Autodesk Inventor part; units mm, degrees
(part 2 of 2)
  line L261 (-632.3012, 486.9524) -> (-657.7012, 472.2877)
  arc A340 (-632.3012, 486.9524) -> (-632.3012, 495.7513) centre (-634.8412, 491.3518) ccw
  arc A341 (-665.3212, 476.6871) -> (-657.7012, 472.2877) centre (-660.2412, 476.6871) ccw
  line L262 (-665.3212, 476.6871) -> (-665.3212, 506.0165)
  arc A342 (-657.7012, 510.4159) -> (-665.3212, 506.0165) centre (-660.2412, 506.0165) ccw
  line L263 (-703.1037, 495.7513) -> (-677.7037, 510.4159)
  line L264 (-670.0837, 506.0165) -> (-670.0837, 476.6871)
  arc A343 (-670.0837, 506.0165) -> (-677.7037, 510.4159) centre (-675.1637, 506.0165) ccw
  arc A344 (-677.7037, 472.2877) -> (-670.0837, 476.6871) centre (-675.1637, 476.6871) ccw
  line L265 (-677.7037, 472.2877) -> (-703.1037, 486.9524)
  arc A345 (-703.1037, 495.7513) -> (-703.1037, 486.9524) centre (-700.5637, 491.3518) ccw
  line L266 (-713.105, 449.0992) -> (-713.105, 478.4286)
  line L267 (-705.485, 482.828) -> (-680.085, 468.1633)
  arc A346 (-705.485, 482.828) -> (-713.105, 478.4286) centre (-708.025, 478.4286) ccw
  arc A347 (-680.085, 459.3645) -> (-680.085, 468.1633) centre (-682.625, 463.7639) ccw
  line L268 (-680.085, 459.3645) -> (-705.485, 444.6998)
  arc A348 (-713.105, 449.0992) -> (-705.485, 444.6998) centre (-708.025, 449.0992) ccw
  line L269 (-677.7038, 417.1118) -> (-703.1038, 431.7765)
  line L270 (-703.1038, 440.5753) -> (-677.7038, 455.24)
  arc A349 (-703.1038, 440.5753) -> (-703.1038, 431.7765) centre (-700.5638, 436.1759) ccw
  arc A350 (-670.0838, 450.8406) -> (-677.7038, 455.24) centre (-675.1638, 450.8406) ccw
  line L271 (-670.0838, 450.8406) -> (-670.0838, 421.5112)
  arc A351 (-677.7038, 417.1118) -> (-670.0838, 421.5112) centre (-675.1638, 421.5112) ccw
  circle A352 centre (-524.3512, 215.4722) radius 9.8425 construction
  line L272 (-511.9687, 219.8716) -> (-486.5687, 234.5363)
  arc A353 (-478.9487, 230.1369) -> (-486.5687, 234.5363) centre (-484.0287, 230.1369) ccw
  line L273 (-478.9487, 230.1369) -> (-478.9487, 200.8075)
  arc A354 (-486.5687, 196.4081) -> (-478.9487, 200.8075) centre (-484.0287, 200.8075) ccw
  line L274 (-486.5687, 196.4081) -> (-511.9687, 211.0728)
  arc A355 (-511.9687, 219.8716) -> (-511.9687, 211.0728) centre (-509.4287, 215.4722) ccw
  line L275 (-521.97, 228.3955) -> (-521.97, 257.7249)
  arc A356 (-514.35, 262.1243) -> (-521.97, 257.7249) centre (-516.89, 257.7249) ccw
  line L276 (-514.35, 262.1243) -> (-488.95, 247.4596)
  arc A357 (-488.95, 238.6608) -> (-488.95, 247.4596) centre (-491.49, 243.0602) ccw
  line L277 (-488.95, 238.6608) -> (-514.35, 223.9961)
  arc A358 (-521.97, 228.3955) -> (-514.35, 223.9961) centre (-516.89, 228.3955) ccw
  line L278 (-534.3525, 223.9961) -> (-559.7525, 238.6608)
  arc A359 (-559.7525, 247.4596) -> (-559.7525, 238.6608) centre (-557.2125, 243.0602) ccw
  line L279 (-559.7525, 247.4596) -> (-534.3525, 262.1243)
  arc A360 (-526.7325, 257.7249) -> (-534.3525, 262.1243) centre (-531.8125, 257.7249) ccw
  line L280 (-526.7325, 257.7249) -> (-526.7325, 228.3955)
  arc A361 (-534.3525, 223.9961) -> (-526.7325, 228.3955) centre (-531.8125, 228.3955) ccw
  line L281 (-536.7338, 211.0728) -> (-562.1338, 196.4081)
  arc A362 (-569.7538, 200.8075) -> (-562.1338, 196.4081) centre (-564.6738, 200.8075) ccw
  line L282 (-569.7538, 200.8075) -> (-569.7538, 230.1369)
  arc A363 (-562.1338, 234.5363) -> (-569.7538, 230.1369) centre (-564.6738, 230.1369) ccw
  line L283 (-562.1338, 234.5363) -> (-536.7338, 219.8716)
  arc A364 (-536.7338, 211.0728) -> (-536.7338, 219.8716) centre (-539.2738, 215.4722) ccw
  line L284 (-526.7325, 202.549) -> (-526.7325, 173.2196)
  arc A365 (-534.3525, 168.8202) -> (-526.7325, 173.2196) centre (-531.8125, 173.2196) ccw
  line L285 (-534.3525, 168.8202) -> (-559.7525, 183.4849)
  arc A366 (-559.7525, 192.2837) -> (-559.7525, 183.4849) centre (-557.2125, 187.8843) ccw
  line L286 (-559.7525, 192.2837) -> (-534.3525, 206.9484)
  arc A367 (-526.7325, 202.549) -> (-534.3525, 206.9484) centre (-531.8125, 202.549) ccw
  circle A368 centre (-524.3512, 270.6482) radius 9.8425 construction
  line L287 (-478.9488, 285.3129) -> (-478.9488, 255.9835)
  arc A369 (-478.9488, 285.3129) -> (-486.5688, 289.7123) centre (-484.0288, 285.3129) ccw
  arc A370 (-486.5688, 251.5841) -> (-478.9488, 255.9835) centre (-484.0288, 255.9835) ccw
  line L288 (-486.5688, 251.5841) -> (-511.9688, 266.2487)
  arc A371 (-511.9688, 275.0476) -> (-511.9688, 266.2487) centre (-509.4288, 270.6482) ccw
  line L289 (-511.9688, 275.0476) -> (-486.5688, 289.7123)
  circle A372 centre (-524.3512, 270.6482) radius 9.8425 construction
  line L290 (-514.35, 317.3002) -> (-488.95, 302.6355)
  arc A373 (-514.35, 317.3002) -> (-521.97, 312.9008) centre (-516.89, 312.9008) ccw
  arc A374 (-488.95, 293.8367) -> (-488.95, 302.6355) centre (-491.49, 298.2361) ccw
  line L291 (-488.95, 293.8367) -> (-514.35, 279.172)
  arc A375 (-521.97, 283.5714) -> (-514.35, 279.172) centre (-516.89, 283.5714) ccw
  line L292 (-521.97, 283.5714) -> (-521.97, 312.9008)
  circle A376 centre (-524.3512, 270.6482) radius 9.8425 construction
  line L293 (-559.7525, 302.6355) -> (-534.3525, 317.3002)
  arc A377 (-559.7525, 302.6355) -> (-559.7525, 293.8367) centre (-557.2125, 298.2361) ccw
  arc A378 (-526.7325, 312.9008) -> (-534.3525, 317.3002) centre (-531.8125, 312.9008) ccw
  line L294 (-526.7325, 312.9008) -> (-526.7325, 283.5714)
  arc A379 (-534.3525, 279.172) -> (-526.7325, 283.5714) centre (-531.8125, 283.5714) ccw
  line L295 (-534.3525, 279.172) -> (-559.7525, 293.8367)
  circle A380 centre (-524.3512, 270.6482) radius 9.8425 construction
  line L296 (-569.7537, 255.9835) -> (-569.7537, 285.3129)
  arc A381 (-569.7537, 255.9835) -> (-562.1337, 251.5841) centre (-564.6737, 255.9835) ccw
  arc A382 (-562.1337, 289.7123) -> (-569.7537, 285.3129) centre (-564.6737, 285.3129) ccw
  line L297 (-562.1337, 289.7123) -> (-536.7337, 275.0476)
  arc A383 (-536.7337, 266.2487) -> (-536.7337, 275.0476) centre (-539.2737, 270.6482) ccw
  line L298 (-536.7337, 266.2487) -> (-562.1337, 251.5841)
  circle A384 centre (-524.3512, 270.6482) radius 9.8425 construction
  line L299 (-534.3525, 223.9961) -> (-559.7525, 238.6608)
  arc A385 (-534.3525, 223.9961) -> (-526.7325, 228.3955) centre (-531.8125, 228.3955) ccw
  arc A386 (-559.7525, 247.4596) -> (-559.7525, 238.6608) centre (-557.2125, 243.0602) ccw
  line L300 (-559.7525, 247.4596) -> (-534.3525, 262.1243)
  arc A387 (-526.7325, 257.7249) -> (-534.3525, 262.1243) centre (-531.8125, 257.7249) ccw
  line L301 (-526.7325, 257.7249) -> (-526.7325, 228.3955)
  circle A388 centre (-524.3512, 270.6482) radius 9.8425 construction
  circle A389 centre (-572.135, 243.0602) radius 9.8425 construction
  circle A390 centre (-619.9187, 270.6482) radius 9.8425 construction
  line L302 (-574.5162, 285.3129) -> (-574.5162, 255.9835)
  arc A391 (-582.1362, 251.5841) -> (-574.5162, 255.9835) centre (-579.5962, 255.9835) ccw
  arc A392 (-607.5362, 275.0476) -> (-607.5362, 266.2487) centre (-604.9962, 270.6482) ccw
  line L303 (-582.1362, 251.5841) -> (-607.5362, 266.2487)
  line L304 (-607.5362, 275.0476) -> (-582.1362, 289.7123)
  arc A393 (-574.5162, 285.3129) -> (-582.1362, 289.7123) centre (-579.5962, 285.3129) ccw
  line L305 (-609.9175, 317.3002) -> (-584.5175, 302.6355)
  arc A394 (-584.5175, 293.8367) -> (-584.5175, 302.6355) centre (-587.0575, 298.2361) ccw
  arc A395 (-617.5375, 283.5714) -> (-609.9175, 279.172) centre (-612.4575, 283.5714) ccw
  line L306 (-584.5175, 293.8367) -> (-609.9175, 279.172)
  line L307 (-617.5375, 283.5714) -> (-617.5375, 312.9008)
  arc A396 (-609.9175, 317.3002) -> (-617.5375, 312.9008) centre (-612.4575, 312.9008) ccw
  line L308 (-655.32, 302.6355) -> (-629.92, 317.3002)
  arc A397 (-622.3, 312.9008) -> (-629.92, 317.3002) centre (-627.38, 312.9008) ccw
  arc A398 (-629.92, 279.172) -> (-622.3, 283.5714) centre (-627.38, 283.5714) ccw
  line L309 (-622.3, 312.9008) -> (-622.3, 283.5714)
  line L310 (-629.92, 279.172) -> (-655.32, 293.8367)
  arc A399 (-655.32, 302.6355) -> (-655.32, 293.8367) centre (-652.78, 298.2361) ccw
  line L311 (-665.3213, 255.9835) -> (-665.3212, 285.3129)
  arc A400 (-657.7013, 289.7123) -> (-665.3212, 285.3129) centre (-660.2413, 285.3129) ccw
  arc A401 (-632.3012, 266.2487) -> (-632.3013, 275.0476) centre (-634.8412, 270.6482) ccw
  line L312 (-657.7013, 289.7123) -> (-632.3013, 275.0476)
  line L313 (-632.3012, 266.2487) -> (-657.7013, 251.5841)
  arc A402 (-665.3213, 255.9835) -> (-657.7013, 251.5841) centre (-660.2413, 255.9835) ccw
  line L314 (-629.92, 223.9961) -> (-655.32, 238.6608)
  arc A403 (-655.32, 247.4596) -> (-655.32, 238.6608) centre (-652.78, 243.0602) ccw
  arc A404 (-622.3, 257.7249) -> (-629.92, 262.1243) centre (-627.38, 257.7249) ccw
  line L315 (-655.32, 247.4596) -> (-629.92, 262.1243)
  line L316 (-622.3, 257.7249) -> (-622.3, 228.3955)
  arc A405 (-629.92, 223.9961) -> (-622.3, 228.3955) centre (-627.38, 228.3955) ccw
  circle A406 centre (-572.135, 298.2361) radius 9.8425 construction
  circle A407 centre (-619.9187, 325.8241) radius 9.8425 construction
  circle A408 centre (-476.5675, 298.2361) radius 9.8425 construction
  circle A409 centre (-476.5675, 353.412) radius 9.8425 construction
  circle A410 centre (-524.3512, 325.8241) radius 9.8425 construction
  line L317 (-514.35, 317.3002) -> (-488.95, 302.6355)
  arc A411 (-488.95, 293.8367) -> (-488.95, 302.6355) centre (-491.49, 298.2361) ccw
  line L318 (-488.95, 293.8367) -> (-514.35, 279.172)
  arc A412 (-521.97, 283.5714) -> (-514.35, 279.172) centre (-516.89, 283.5714) ccw
  line L319 (-521.97, 283.5714) -> (-521.97, 312.9008)
  arc A413 (-514.35, 317.3002) -> (-521.97, 312.9008) centre (-516.89, 312.9008) ccw
  line L320 (-511.9687, 330.2235) -> (-486.5687, 344.8882)
  arc A414 (-478.9487, 340.4888) -> (-486.5687, 344.8882) centre (-484.0287, 340.4888) ccw
  line L321 (-478.9487, 340.4888) -> (-478.9487, 311.1594)
  arc A415 (-486.5687, 306.76) -> (-478.9487, 311.1594) centre (-484.0287, 311.1594) ccw
  line L322 (-486.5687, 306.76) -> (-511.9687, 321.4247)
  arc A416 (-511.9687, 330.2235) -> (-511.9687, 321.4247) centre (-509.4287, 325.8241) ccw
  line L323 (-521.97, 338.7473) -> (-521.97, 368.0767)
  arc A417 (-514.35, 372.4761) -> (-521.97, 368.0767) centre (-516.89, 368.0767) ccw
  line L324 (-514.35, 372.4761) -> (-488.95, 357.8114)
  arc A418 (-488.95, 349.0126) -> (-488.95, 357.8114) centre (-491.49, 353.412) ccw
  line L325 (-488.95, 349.0126) -> (-514.35, 334.3479)
  arc A419 (-521.97, 338.7473) -> (-514.35, 334.3479) centre (-516.89, 338.7473) ccw
  line L326 (-534.3525, 334.3479) -> (-559.7525, 349.0126)
  arc A420 (-559.7525, 357.8114) -> (-559.7525, 349.0126) centre (-557.2125, 353.412) ccw
  line L327 (-559.7525, 357.8114) -> (-534.3525, 372.4761)
  arc A421 (-526.7325, 368.0767) -> (-534.3525, 372.4761) centre (-531.8125, 368.0767) ccw
  line L328 (-526.7325, 368.0767) -> (-526.7325, 338.7473)
  arc A422 (-534.3525, 334.3479) -> (-526.7325, 338.7473) centre (-531.8125, 338.7473) ccw
  line L329 (-536.7338, 321.4247) -> (-562.1338, 306.76)
  arc A423 (-569.7538, 311.1594) -> (-562.1338, 306.76) centre (-564.6738, 311.1594) ccw
  line L330 (-569.7538, 311.1594) -> (-569.7538, 340.4888)
  arc A424 (-562.1338, 344.8882) -> (-569.7538, 340.4888) centre (-564.6738, 340.4888) ccw
  line L331 (-562.1338, 344.8882) -> (-536.7338, 330.2235)
  arc A425 (-536.7338, 321.4247) -> (-536.7338, 330.2235) centre (-539.2738, 325.8241) ccw
  line L332 (-574.5163, 340.4888) -> (-574.5163, 311.1594)
  arc A426 (-582.1363, 306.76) -> (-574.5163, 311.1594) centre (-579.5963, 311.1594) ccw
  line L333 (-582.1363, 306.76) -> (-607.5363, 321.4247)
  arc A427 (-607.5363, 330.2235) -> (-607.5363, 321.4247) centre (-604.9963, 325.8241) ccw
  line L334 (-607.5363, 330.2235) -> (-582.1363, 344.8882)
  arc A428 (-574.5163, 340.4888) -> (-582.1363, 344.8882) centre (-579.5963, 340.4888) ccw
  line L335 (-609.9175, 372.4761) -> (-584.5175, 357.8114)
  arc A429 (-584.5175, 349.0126) -> (-584.5175, 357.8114) centre (-587.0575, 353.412) ccw
  line L336 (-584.5175, 349.0126) -> (-609.9175, 334.3479)
  arc A430 (-617.5375, 338.7473) -> (-609.9175, 334.3479) centre (-612.4575, 338.7473) ccw
  line L337 (-617.5375, 338.7473) -> (-617.5375, 368.0767)
  arc A431 (-609.9175, 372.4761) -> (-617.5375, 368.0767) centre (-612.4575, 368.0767) ccw
  line L338 (-655.32, 357.8114) -> (-629.92, 372.4761)
  arc A432 (-622.3, 368.0767) -> (-629.92, 372.4761) centre (-627.38, 368.0767) ccw
  line L339 (-622.3, 368.0767) -> (-622.3, 338.7473)
  arc A433 (-629.92, 334.3479) -> (-622.3, 338.7473) centre (-627.38, 338.7473) ccw
  line L340 (-629.92, 334.3479) -> (-655.32, 349.0126)
  arc A434 (-655.32, 357.8114) -> (-655.32, 349.0126) centre (-652.78, 353.412) ccw
  line L341 (-665.3212, 311.1594) -> (-665.3212, 340.4888)
  arc A435 (-657.7012, 344.8882) -> (-665.3212, 340.4888) centre (-660.2412, 340.4888) ccw
  line L342 (-657.7012, 344.8882) -> (-632.3012, 330.2235)
  arc A436 (-632.3012, 321.4247) -> (-632.3012, 330.2235) centre (-634.8412, 325.8241) ccw
  line L343 (-632.3012, 321.4247) -> (-657.7012, 306.76)
  arc A437 (-665.3212, 311.1594) -> (-657.7012, 306.76) centre (-660.2412, 311.1594) ccw
  line L344 (-629.92, 279.172) -> (-655.32, 293.8367)
  arc A438 (-655.32, 302.6355) -> (-655.32, 293.8367) centre (-652.78, 298.2361) ccw
  line L345 (-655.32, 302.6355) -> (-629.92, 317.3002)
  arc A439 (-622.3, 312.9008) -> (-629.92, 317.3002) centre (-627.38, 312.9008) ccw
  line L346 (-622.3, 312.9008) -> (-622.3, 283.5714)
  arc A440 (-629.92, 279.172) -> (-622.3, 283.5714) centre (-627.38, 283.5714) ccw
  point P0 (0, 0)
  point P1 (-396.9279, 381)
  point P2 (-383.3812, 357.5365)
  point P3 (-424.0213, 381)
  point P4 (-383.3812, 404.4635)
  point P5 (-385.7625, 408.588)
  point P6 (-426.4025, 385.1244)
  point P7 (-426.4025, 432.0515)
  point P8 (-431.165, 432.0515)
  point P9 (-431.165, 385.1244)
  point P10 (-471.805, 408.588)
  point P11 (-474.1862, 404.4635)
  point P12 (-433.5462, 381)
  point P13 (-474.1862, 357.5365)
  point P14 (-471.805, 353.412)
  point P15 (-431.165, 376.8756)
  point P16 (-431.165, 329.9485)
  point P17 (-426.4025, 329.9485)
  point P18 (-426.4025, 376.8756)
  point P19 (-385.7625, 353.412)
  point P20 (-445.8825, 368.3784)
  point P21 (-474.1862, 302.3606)
  point P22 (-433.5462, 325.8241)
  point P23 (-474.1862, 349.2876)
  point P24 (-474.1862, 332.2933)
  point P25 (-431.165, 274.7726)
  point P26 (-431.165, 321.6996)
  point P27 (-471.805, 298.2361)
  point P28 (-457.0875, 289.739)
  point P29 (-385.7625, 298.2361)
  point P30 (-426.4025, 321.6996)
  point P31 (-426.4025, 274.7726)
  point P32 (-411.685, 283.2698)
  point P33 (-383.3812, 349.2876)
  point P34 (-424.0212, 325.8241)
  point P35 (-383.3812, 302.3606)
  point P36 (-383.3812, 319.3549)
  point P37 (-426.4025, 376.8756)
  point P38 (-426.4025, 329.9485)
  point P39 (-385.7625, 353.412)
  point P40 (-400.48, 361.9092)
  point P41 (-433.5462, 270.6482)
  point P42 (-474.1862, 294.1117)
  point P43 (-474.1862, 247.1846)
  point P44 (-459.4687, 255.6818)
  point P45 (-431.165, 266.5237)
  point P46 (-471.805, 243.0602)
  point P47 (-431.165, 219.5967)
  point P48 (-431.165, 236.591)
  point P49 (-426.4025, 266.5237)
  point P50 (-426.4025, 219.5967)
  point P51 (-385.7625, 243.0602)
  point P52 (-400.48, 251.5574)
  point P53 (-424.0212, 270.6482)
  point P54 (-383.3812, 247.1846)
  point P55 (-383.3812, 294.1117)
  point P56 (-398.0988, 285.6145)
  point P57 (-426.4025, 274.7726)
  point P58 (-385.7625, 298.2361)
  point P59 (-426.4025, 321.6996)
  point P60 (-426.4025, 304.7053)
  point P61 (-448.2638, 223.9694)
  point P62 (-474.1862, 238.9357)
  point P63 (-433.5462, 215.4722)
  point P64 (-474.1862, 192.0087)
  point P65 (-445.8825, 202.8506)
  point P66 (-471.805, 187.8843)
  point P67 (-431.165, 211.3478)
  point P68 (-431.165, 164.4208)
  point P69 (-426.4025, 194.3535)
  point P70 (-426.4025, 164.4208)
  point P71 (-426.4025, 211.3478)
  point P72 (-385.7625, 187.8843)
  point P73 (-409.3037, 206.9751)
  point P74 (-383.3812, 192.0087)
  point P75 (-424.0212, 215.4722)
  point P76 (-383.3812, 238.9357)
  point P77 (-411.685, 228.0938)
  point P78 (-385.7625, 243.0602)
  point P79 (-426.4025, 219.5967)
  point P80 (-426.4025, 266.5237)
  point P81 (-474.1862, 136.8328)
  point P82 (-433.5462, 160.2963)
  point P83 (-474.1862, 183.7598)
  point P84 (-474.1862, 166.7655)
  point P85 (-431.165, 109.2448)
  point P86 (-431.165, 156.1719)
  point P87 (-471.805, 132.7084)
  point P88 (-457.0875, 124.2112)
  point P89 (-385.7625, 132.7084)
  point P90 (-426.4025, 156.1719)
  point P91 (-426.4025, 109.2448)
  point P92 (-411.685, 117.742)
  point P93 (-383.3812, 183.7598)
  point P94 (-424.0212, 160.2963)
  point P95 (-383.3812, 136.8328)
  point P96 (-383.3812, 153.8271)
  point P97 (-426.4025, 211.3478)
  point P98 (-426.4025, 164.4208)
  point P99 (-385.7625, 187.8843)
  point P100 (-400.48, 196.3814)
  point P101 (-431.165, 156.1719)
  point P102 (-431.165, 109.2448)
  point P103 (-431.165, 126.2392)
  point P104 (-471.805, 132.7084)
  point P105 (-474.1862, 128.5839)
  point P106 (-433.5462, 105.1204)
  point P107 (-448.2638, 113.6175)
  point P108 (-474.1862, 81.6569)
  point P109 (-471.805, 77.5324)
  point P110 (-431.165, 100.9959)
  point P111 (-445.8825, 92.4988)
  point P112 (-431.165, 54.0689)
  point P113 (-426.4025, 54.0689)
  point P114 (-426.4025, 100.9959)
  point P115 (-426.4025, 84.0016)
  point P116 (-385.7625, 77.5324)
  point P117 (-383.3812, 81.6569)
  point P118 (-424.0212, 105.1204)
  point P119 (-409.3037, 96.6232)
  point P120 (-383.3812, 128.5839)
  point P121 (-383.3812, 73.408)
  point P122 (-424.0212, 49.9445)
  point P123 (-383.3812, 26.481)
  point P124 (-383.3812, 43.4753)
  point P125 (-474.1862, 26.481)
  point P126 (-433.5462, 49.9445)
  point P127 (-474.1862, 73.408)
  point P128 (-474.1862, 56.4137)
  point P129 (-519.5887, 105.1204)
  point P130 (-478.9487, 81.6569)
  point P131 (-478.9487, 128.5839)
  point P132 (-493.6663, 120.0867)
  point P133 (-521.97, 54.0689)
  point P134 (-481.33, 77.5324)
  point P135 (-521.97, 100.9959)
  point P136 (-521.97, 84.0016)
  point P137 (-478.9487, 26.481)
  point P138 (-478.9487, 73.408)
  point P139 (-519.5887, 49.9445)
  point P140 (-504.8712, 41.4473)
  point P141 (-433.5462, 49.9445)
  point P142 (-474.1862, 73.408)
  point P143 (-474.1862, 26.481)
  point P144 (-459.4687, 34.9781)
  point P145 (-431.165, 100.9959)
  point P146 (-471.805, 77.5324)
  point P147 (-431.165, 54.0689)
  point P148 (-431.165, 71.0632)
  point P149 (-478.9487, 136.8328)
  point P150 (-519.5887, 160.2963)
  point P151 (-504.8712, 151.7992)
  point P152 (-478.9487, 183.7598)
  point P153 (-481.33, 132.7084)
  point P154 (-521.97, 109.2448)
  point P155 (-507.2525, 117.742)
  point P156 (-521.97, 156.1719)
  point P157 (-478.9487, 128.5839)
  point P158 (-478.9487, 81.6569)
  point P159 (-478.9487, 98.6512)
  point P160 (-519.5887, 105.1204)
  point P161 (-474.1862, 128.5839)
  point P162 (-433.5462, 105.1204)
  point P163 (-448.2638, 113.6175)
  point P164 (-474.1862, 81.6569)
  point P165 (-471.805, 132.7084)
  point P166 (-431.165, 156.1719)
  point P167 (-445.8825, 147.6747)
  point P168 (-431.165, 109.2448)
  point P169 (-478.9487, 81.6569)
  point P170 (-519.5887, 105.1204)
  point P171 (-504.8712, 96.6232)
  point P172 (-478.9487, 128.5839)
  point P173 (-481.33, 132.7084)
  point P174 (-521.97, 109.2448)
  point P175 (-507.2525, 117.742)
  point P176 (-521.97, 156.1719)
  point P177 (-526.7325, 156.1719)
  point P178 (-526.7325, 109.2448)
  point P179 (-526.7325, 126.2392)
  point P180 (-567.3725, 132.7084)
  point P181 (-529.1137, 160.2963)
  point P182 (-569.7537, 136.8328)
  point P183 (-569.7537, 183.7598)
  point P184 (-543.8313, 168.7935)
  point P185 (-574.5162, 183.7598)
  point P186 (-574.5162, 136.8328)
  point P187 (-615.1562, 160.2963)
  point P188 (-589.2338, 175.2627)
  point P189 (-567.3725, 132.7084)
  point P190 (-526.7325, 156.1719)
  point P191 (-541.45, 147.6747)
  point P192 (-526.7325, 109.2448)
  point P193 (-521.97, 109.2448)
  point P194 (-521.97, 156.1719)
  point P195 (-521.97, 139.1775)
  point P196 (-481.33, 132.7084)
  point P197 (-478.9487, 136.8328)
  point P198 (-519.5887, 160.2963)
  point P199 (-504.8712, 151.7992)
  dimension "d168" = 5.08
  dimension "d169" = 25.4
  dimension "d172" = 360
  dimension "d177" = 10.16
  dimension "d179" = 381
  dimension "d183" = 360
  dimension "d185" = 10.16
  dimension "d186" = 25.4
  dimension "d189" = 360
  dimension "d193" = 360
  dimension "d197" = 360
  dimension "d201" = 360
  dimension "d205" = 120
  dimension "d209" = 60
  dimension "d211" = 4.7625
  dimension "d212" = 9.6375
  dimension "d213" = 2.3813
  dimension "d214" = 12.6077
  dimension "d216" = 368.9958
  dimension "d219" = 360
  dimension "d223" = 360
  dimension "d227" = 180
  dimension "d231" = 120
  dimension "d235" = 360
  dimension "d239" = 360
  dimension "d243" = 120
  dimension "d247" = 120
  dimension "d251" = 120
  dimension "d255" = 360
  dimension "d259" = 360
  dimension "d263" = 360
  dimension "d267" = 360
  dimension "d271" = 360
  dimension "d275" = 360
  dimension "d279" = 360
  dimension "d283" = 360
  dimension "d287" = 360
  constraints: 752 point on line, 670 end point, 648 point on circle, 373 centre point, 55 tangent, 27 equal radius, 8 coincident, 4 horizontal alignment, 3 midpoint, 1 perpendicular, 1 vertical, 2470 other
  measures "d168" radius of A1
  measures "d169" horizontal distance of A1.centre A2.centre
  measures "d177" diameter of A24
  measures "d179" distance of L23.start L23.end
  measures "d185" diameter of A42
  measures "d186" distance between parallel lines of L46 L48
  measures "d211" distance between parallel lines of L15 L17
  measures "d212" horizontal distance of A17.centre point (-445.883, 368.378)
  measures "d213" distance between parallel lines of L3 L7
  measures "d214" diameter of A25
  measures "d216" distance of L24.start L24.end
body "Solid1"
